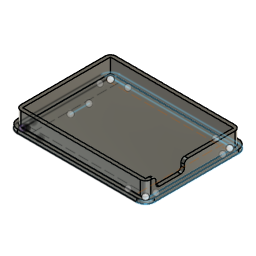
scamp-oled-case-base v3 (Autodesk Fusion 360 design; units mm, degrees)
Autodesk Fusion 360 part; units mm, degrees
sketch "Sketch1" plane through (0, 0, 0) normal (0, 0, 1) x (1, 0, 0)
  line L0 (1, 0) -> (69, 0)
  line L1 (70, 1) -> (70, 49)
  line L2 (69, 50) -> (1, 50)
  line L3 (0, 49) -> (0, 1)
  line L4 (0, 2.5) -> (70, 2.5) construction
  line L5 (0, 47.5) -> (70, 47.5) construction
  line L6 (65, 50) -> (65, 0) construction
  line L7 (5, 50) -> (5, 0) construction
  line L8 (0, 50) -> (10, 50)
  line L9 (0, 44) -> (0, 50)
  line L10 (70, 50) -> (60, 50)
  line L11 (70, 44) -> (70, 50)
  line L12 (0, 0) -> (10, 0)
  line L13 (0, 6) -> (0, 0)
  line L14 (70, 0) -> (60, 0)
  line L15 (70, 6) -> (70, 0)
  line L16 (6.8, 20.5) -> (6.8, 31)
  arc A0 (1, 50) -> (0, 49) centre (1, 49) ccw
  arc A1 (70, 49) -> (69, 50) centre (69, 49) ccw
  arc A2 (0, 1) -> (1, 0) centre (1, 1) ccw
  arc A3 (69, 0) -> (70, 1) centre (69, 1) ccw
  line L17 (72, 1) -> (72, 49)
  arc A4 (72, 49) -> (69, 52) centre (69, 49) ccw
  line L18 (69, 52) -> (1, 52)
  arc A5 (1, 52) -> (-2, 49) centre (1, 49) ccw
  line L19 (-2, 49) -> (-2, 1)
  arc A6 (-2, 1) -> (1, -2) centre (1, 1) ccw
  line L20 (1, -2) -> (69, -2)
  arc A7 (69, -2) -> (72, 1) centre (69, 1) ccw
  line L21 (1, -4) -> (69, -4)
  arc A8 (69, -4) -> (74, 1) centre (69, 1) ccw
  line L22 (74, 1) -> (74, 49)
  arc A9 (74, 49) -> (69, 54) centre (69, 49) ccw
  line L23 (69, 54) -> (1, 54)
  arc A10 (1, 54) -> (-4, 49) centre (1, 49) ccw
  line L24 (-4, 49) -> (-4, 1)
  arc A11 (-4, 1) -> (1, -4) centre (1, 1) ccw
  dimension "d1" = 2
  dimension "d2" = 4
  dimension "d3" = 5
  dimension "d4" = 5
  dimension "d5" = 2.5
  dimension "d6" = 2.5
  dimension "d7" = 10
  dimension "d8" = 6
  dimension "d9" = 10
  dimension "d10" = 6
  dimension "d11" = 10
  dimension "d12" = 6
  dimension "d13" = 10
  dimension "d14" = 6
  dimension "d20" = 10.5
  dimension "d41" = 1
  dimension "d42" = 1
  dimension "d43" = 1
  dimension "d44" = 1
  constraint horizontal L0
  constraint vertical L1
  constraint horizontal L2
  constraint vertical L3
  constraint coincident L12.start L13.end
  constraint coincident L3 L4.start
  constraint perpendicular L3 L4
  constraint coincident L1 L4.end
  constraint coincident L3 L5.start
  constraint perpendicular L3 L5
  constraint coincident L1 L5.end
  constraint coincident L2 L6.start
  constraint perpendicular L2 L6
  constraint coincident L0 L6.end
  constraint coincident L2 L7.start
  constraint perpendicular L2 L7
  constraint coincident L0 L7.end
  constraint horizontal L8
  constraint vertical L9
  constraint horizontal L10
  constraint vertical L11
  constraint horizontal L12
  constraint vertical L13
  constraint horizontal L14
  constraint vertical L15
  constraint vertical L16
  constraint coincident L8.start L3
  constraint coincident L8.start L2
  constraint tangent L3 A0
  constraint tangent L2 A0
  constraint coincident L10.start L2
  constraint coincident L10.start L1
  constraint tangent L2 A1
  constraint tangent L1 A1
  constraint coincident L12.start L3
  constraint coincident L12.start L0
  constraint tangent L3 A2
  constraint tangent L0 A2
  constraint coincident L14.start L1
  constraint coincident L14.start L0
  constraint tangent L1 A3
  constraint tangent L0 A3
  measures "d3" distance of L3 L7
  measures "d4" distance of L1 L6
  measures "d5" distance of L2 L5
  measures "d6" distance of L0 L4
  measures "d7" distance of L8.start L8.end
  measures "d8" distance of L8.start L9.start
  measures "d9" distance of L10.start L10.end
  measures "d10" distance of L10.start L11.start
  measures "d11" distance of L12.start L12.end
  measures "d12" distance of L12.start L13.start
  measures "d13" distance of L14.start L14.end
  measures "d14" distance of L14.start L15.start
  measures "d20" distance of L16.end L16.start
  measures "d41" radius of A0
  measures "d42" radius of A1
  measures "d43" radius of A2
  measures "d44" radius of A3
extrude "Extrude8" add sketch "Sketch1" along normal blind 2 contours L0 L1 L2 L3 L8 L9 L10 L11 L12 L13 L14 L15 A0 A1 A2 A3 | L17 A4 L18 A5 L19 A6 L20 A7 | L21 A8 L22 A9 L23 A10 L24 A11
extrude "Extrude9" add sketch "Sketch1" along normal blind 10 contours L17 A4 L18 A5 L19 A6 L20 A7
sketch "Sketch3" plane through (72, 0, 0) normal (1, 0, 0) x (0, 1, 0)
  line L0 (1, 2) -> (49, 2)
  line L1 (49, 2) -> (49, 10)
  line L2 (49, 10) -> (1, 10)
  line L3 (1, 10) -> (1, 2)
  line L4 (12, 10) -> (12, 0) construction
  line L5 (-4, 0) -> (-4, 2)
  line L6 (3.9489, 10) -> (20.1491, 10)
  line L7 (20.1491, 10) -> (20.1491, 4.2646)
  line L8 (20.1491, 4.2646) -> (3.9489, 4.2646)
  line L9 (3.9489, 4.2646) -> (3.9489, 10)
  dimension "d58" = 16
  constraint coincident L2 L4.start
  constraint perpendicular L2 L4
  constraint horizontal L6
  constraint vertical L7
  constraint horizontal L8
  constraint vertical L9
  constraint coincident L2 L6.start
  measures "d58" distance of L4 L5
extrude "Extrude10" cut sketch "Sketch3" against normal blind 10 contours L2 L6 L7 L8 L9
fillet "Fillet1" radius 2 1 edges at (71, 3.9489, 10)
fillet "Fillet2" radius 2 1 edges at (71, 20.1491, 10)
fillet "Fillet3" radius 2 1 edges at (71, 20.1491, 4.2646)
fillet "Fillet4" radius 2 1 edges at (71, 3.9489, 4.2646)
